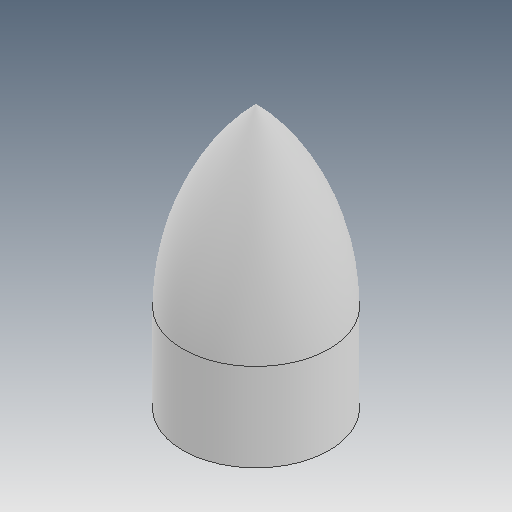
# Autodesk Inventor part: MOTOR SHAFT NUT
Saved by Autodesk Inventor 2020 (Build 240168000, 168)
## iProperties
Created: 2020-04-16
Part Number: MOTOR SHAFT NUT
Material: Generic
Document SubType Name: Modeling
Designer: John K
Density: 1 g/cm^3
Appearance: Default
Description: INCL W/ MOTOR
Author: John K
Autodesk Inventor part; units mm, degrees
ref_plane "YZ Plane" through (0, 0, 0) normal (1, 0, 0) x (0, 1, 0)
ref_plane "XZ Plane" through (0, 0, 0) normal (0, 1, 0) x (-1, 0, 0)
ref_plane "XY Plane" through (0, 0, 0) normal (0, 0, 1) x (1, 0, 0)
sketch "Sketch1" plane through (0, 0, 0) normal (0, 0, 1) x (1, 0, 0)
  line L0 (-2.5, 0) -> (-2.5, 6)
  line L1 (-2.5, 6) -> (0, 6)
  line L2 (0, 6) -> (0, 18)
  line L3 (-5, 6) -> (-5, 0)
  line L4 (-5, 0) -> (-2.5, 0)
  arc A0 (0, 18) -> (-5, 6) centre (11.9, 6) ccw
  line L5 (0, 0) -> (0, -10.9091)
  dimension "d0" = 5
  dimension "d1" = 10
  dimension "d2" = 18
  dimension "d3" = 6
  constraints: 12 end point, 3 perpendicular, 2 point on circle, 2 vertical, 1 centre point, 1 collinear, 1 horizontal alignment, 1 parallel, 1 point on line, 1 tangent
  measures "d0" diameter of L0 L5
  measures "d1" diameter of L3 L5
  measures "d2" distance from line of L2.end L4
  measures "d3" distance of L0.start L0.end
revolve "Revolution1" add sketch "Sketch1" angle 360 about axis through (0, 0, 0) along (0, -1, 0)
body "Solid1"
